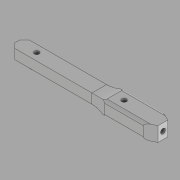
# Autodesk Inventor part: Link_3
Saved by Autodesk Inventor 2020 (Build 240168000, 168)
## iProperties
Created: 2020-02-22
Part Number: Link_3
Material: Generic
Document SubType Name: Modeling
Designer: Pece Jovanovski
Density: 1 g/cm^3
Appearance: Default
Mass: 0.0483013 g
Surface Area: 1.38192 cm^2
Volume: 0.0483013 cm^3
Author: Pece Jovanovski
Autodesk Inventor part; units mm, degrees
ref_plane "YZ Plane" through (0, 0, 0) normal (1, 0, 0) x (0, 1, 0)
ref_plane "XZ Plane" through (0, 0, 0) normal (0, 1, 0) x (-1, 0, 0)
ref_plane "XY Plane" through (0, 0, 0) normal (0, 0, 1) x (1, 0, 0)
sketch "Sketch1" plane through (0, 0, 0) normal (0, 0, 1) x (1, 0, 0)
  line L0 (-8.1593, 0.75) -> (1.3407, 0.75)
  line L1 (1.3407, -0.75) -> (-8.1593, -0.75)
  line L2 (-8.6593, -0.25) -> (-8.6593, 0.25)
  circle A0 centre (-6.6593, 0) radius 0.25
  circle A1 centre (2.3407, 0) radius 0.25
  line L3 (-11.6593, 0) -> (9.3407, 0) projected
  line L4 (1.3407, -0.75) -> (1.3407, -1.0115)
  line L5 (1.3407, 0.75) -> (1.3407, 0.9885)
  line L6 (-8.1593, 0.75) -> (-8.1593, 0.75)
  line L7 (-8.6593, 0.25) -> (-8.6593, 0.25)
  line L8 (-8.1593, -0.75) -> (-8.1593, -0.75)
  line L9 (-8.6593, -0.25) -> (-8.6593, -0.25)
  line L10 (1.3407, 0.9885) -> (5.3407, 0.9885)
  line L11 (6.3407, 0.4885) -> (6.3407, -0.5115)
  line L12 (1.3407, -1.0115) -> (5.3407, -1.0115)
  line L13 (5.3407, -1.0115) -> (6.3407, -0.5115)
  line L14 (5.3407, 0.9885) -> (6.3407, 0.4885)
  line L15 (-8.6593, 0.25) -> (-8.1593, 0.75)
  line L16 (-8.6593, -0.25) -> (-8.1593, -0.75)
  point P0 (0, 0)
  point P1 (-8.6593, 0.75)
  point P2 (-8.6593, -0.75)
  point P3 (6.3407, -1.0115)
  point P4 (6.3407, 0.9885)
  point P5 (-8.6593, 0)
  point P6 (6.3407, 0.9885)
  dimension "d2" = 0.5
  dimension "d4" = 0.5
  dimension "d34" = 9
  dimension "d36" = 1.5
  dimension "d37" = 2
  dimension "d38" = 2
  dimension "d39" = 8
  dimension "d40" = 5
  dimension "d56" = 1
  dimension "d57" = 0.5
  dimension "d58" = 1
  dimension "d59" = 0.5
  dimension "d60" = 0.5
  dimension "d61" = 0.5
  dimension "d62" = 0.5
  dimension "d63" = 0.5
  constraints: 32 end point, 13 point on line, 3 horizontal, 3 horizontal alignment, 2 centre point, 2 collinear, 2 perpendicular, 2 vertical, 1 midpoint, 1 parallel, 1 other
  measures "d2" diameter of A0
  measures "d4" diameter of A1
  measures "d34" distance of A1.centre A0.centre
  measures "d36" distance of point (-8.659, -0.75) point (-8.659, 0.75)
  measures "d37" distance of point (6.341, 0.989) point (6.341, -1.011)
  measures "d38" distance from line of L2 A0.centre
  measures "d39" horizontal distance of L1.start A0.centre
  measures "d40" distance of L5.end point (6.341, 0.989)
  measures "d56" distance of L12.end point (6.341, -1.011)
  measures "d57" distance of L11.end point (6.341, -1.011)
  measures "d58" distance of L10.end point (6.341, 0.989)
  measures "d59" distance of L11.start point (6.341, 0.989)
  measures "d60" distance of L7.end point (-8.659, 0.75)
  measures "d61" distance of L6.end point (-8.659, 0.75)
  measures "d62" distance of L9.end point (-8.659, -0.75)
  measures "d63" distance of L8.start point (-8.659, -0.75)
extrude "Extrusion1" add sketch "Sketch1" along normal mid plane 1 contours L0 L5 L10 L14 L11 L3 A1 A0 L2 L15 | L3 A0 A1 L11 L13 L12 L4 L1 L16 L2
sketch "Sketch2" plane through (0, 0, 0.5) normal (0, 0, 1) x (1, 0, 0)
  circle A0 centre (2.3407, 0) radius 0.25 projected
  circle A1 centre (-6.6593, 0) radius 0.25 projected
  line L0 (1.3407, 0.75) -> (-8.1593, 0.75) projected
  line L1 (-8.6593, 0.25) -> (-8.6593, -0.25) projected
  line L2 (-8.1593, -0.75) -> (1.3407, -0.75) projected
  line L3 (1.3407, 0.75) -> (-8.1593, 0.75) projected
  line L4 (1.3407, 0.75) -> (1.3407, -0.75)
  line L5 (1.3407, -0.75) -> (1.3407, -1.0115) projected
  line L6 (1.3407, 0.9885) -> (1.3407, 0.75) projected
  line L7 (1.3407, -1.0115) -> (5.3407, -1.0115) projected
  line L8 (5.3407, -1.0115) -> (6.3407, -0.5115) projected
  line L9 (6.3407, -0.5115) -> (6.3407, 0.4885) projected
  line L10 (6.3407, 0.4885) -> (5.3407, 0.9885) projected
  line L11 (5.3407, 0.9885) -> (1.3407, 0.9885) projected
  line L12 (-8.1593, 0.75) -> (-8.6593, 0.25) projected
  line L13 (-8.6593, -0.25) -> (-8.1593, -0.75) projected
  point P0 (0, 0)
  point P1 (-8.6593, 0.75)
  constraints: 2 end point, 1 perpendicular
extrude "Extrusion2" add sketch "Sketch2" along normal blind 0.25 contours L6 L11 L10 L9 L8 L7 L5 L4
sketch "Sketch3" plane through (0, 0, -0.5) normal (0, 0, -1) x (-1, 0, 0)
  circle A0 centre (-2.3407, 0) radius 0.25 projected
  circle A1 centre (6.6593, 0) radius 0.25 projected
  line L0 (8.1593, 0.75) -> (-1.3407, 0.75) projected
  line L1 (-1.3407, -0.75) -> (8.1593, -0.75) projected
  line L2 (8.6593, -0.25) -> (8.6593, 0.25) projected
  line L3 (-0.3407, -0.75) -> (-0.3407, 0.75) projected
  line L4 (8.1593, -0.75) -> (-1.3407, -0.75) projected
  line L5 (-1.3407, 0.75) -> (-1.3407, -0.75)
  line L6 (-1.3407, 0.75) -> (-1.3407, 0.9885) projected
  line L7 (-1.3407, -1.0115) -> (-1.3407, -0.75) projected
  line L8 (8.1593, -0.75) -> (8.6593, -0.25) projected
  line L9 (8.6593, 0.25) -> (8.1593, 0.75) projected
  line L10 (-1.3407, 0.9885) -> (-5.3407, 0.9885) projected
  line L11 (-5.3407, 0.9885) -> (-6.3407, 0.4885) projected
  line L12 (-6.3407, 0.4885) -> (-6.3407, -0.5115) projected
  line L13 (-6.3407, -0.5115) -> (-5.3407, -1.0115) projected
  line L14 (-5.3407, -1.0115) -> (-1.3407, -1.0115) projected
  point P0 (0, 0)
  point P1 (8.6593, -0.75)
  constraints: 2 end point, 1 perpendicular, 1 vertical alignment
extrude "Extrusion3" add sketch "Sketch3" along normal blind 0.25 contours L5 L7 L14 L13 L12 L11 L10 L6
fillet "Fillet5" radius 5 4 edges at (1.3407, 0, 0.5) (1.3407, 0.75, 0) (1.3407, -0.75, 0) (1.3407, 0, -0.5)
sketch "Sketch10" plane through (0, 0, -0.75) normal (0, 0, -1) x (-1, 0, 0)
  circle A0 centre (-2.3407, 0) radius 0.25 projected
  circle A1 centre (-2.3407, 0) radius 0.375
  circle A2 centre (-2.3407, 0) radius 0.5
  point P0 (0, 0)
  dimension "d48" = 0.75
  dimension "d49" = 1
  constraints: 2 centre point, 2 coincident
  measures "d48" diameter of A1
  measures "d49" diameter of A2
extrude "Extrusion10" add sketch "Sketch10" along normal blind 0.15 contours A1
chamfer "Chamfer1" distance 0.1 angle 45 1 edges at (2.7157, 0, -0.75) measured on face at (3.2157, 0, -0.75)
fillet "Fillet6" radius 0.25 1 edges at (3.3407, 0.9885, -0.75)
fillet "Fillet7" radius 0.25 3 edges at (3.3407, -1.0115, -0.75) (3.3407, -1.0115, 0.75) (3.3407, 0.9885, 0.75)
sketch "Sketch12" plane through (0, 0, -0.5) normal (0, 0, -1) x (-1, 0, 0)
  circle A0 centre (6.6593, 0) radius 0.25 projected
  circle A1 centre (6.6593, 0) radius 0.625
  circle A2 centre (6.6593, 0) radius 0.375
  point P0 (0, 0)
  dimension "d66" = 1.25
  dimension "d67" = 0.75
  constraints: 2 centre point, 2 coincident
  measures "d66" diameter of A1
  measures "d67" diameter of A2
extrude "Extrusion11" add sketch "Sketch12" along normal blind 0.25 contours A2
extrude "Extrusion12" add sketch "Sketch12" along normal blind 0.15 contours A1
fillet "Fillet8" radius 0.25 1 edges at (-6.2843, 0, -0.65)
fillet "Fillet9" radius 0.1 1 edges at (-6.0343, 0, -0.5)
sketch "Sketch14" plane through (6.3407, -0.5115, 0.75) normal (1, 0, 0) x (0, 0, -1)
  circle A0 centre (0.75, 0.5115) radius 0.25
  dimension "d77" = 0.5
  constraints: 1 centre point, 1 coincident
  measures "d77" diameter of A0
extrude "Extrusion13" cut sketch "Sketch14" against normal blind 3
equation "\"d62\" = d60"
equation "\"d63\" = d61"
body "Solid1"
